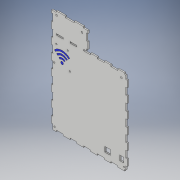
# Autodesk Inventor part: 9 zijplaat met RFID
Saved by Autodesk Inventor 2019 (Build 230136000, 136)
## iProperties
Created: 2021-01-22
Part Number: 9 zijplaat met RFID
Material: Generic
Document SubType Name: Sheet Metal
Designer: Stefan
Density: 1 g/cm^3
Sheet Metal Rule: Default_mm
Appearance: Default
Author: Stefan
Autodesk Inventor part; units mm, degrees
ref_plane "YZ Plane" through (0, 0, 0) normal (1, 0, 0) x (0, 1, 0)
ref_plane "XZ Plane" through (0, 0, 0) normal (0, 1, 0) x (-1, 0, 0)
ref_plane "XY Plane" through (0, 0, 0) normal (0, 0, 1) x (1, 0, 0)
sketch "Sketch1" plane through (0, 0, 0) normal (0, 0, 1) x (1, 0, 0)
  line L0 (-80, -90.5) -> (80, -90.5)
  line L1 (80, -90.5) -> (80, 90.5)
  line L2 (80, 90.5) -> (-80, 90.5)
  line L3 (-80, 90.5) -> (-80, -90.5)
  line L4 (-80, -90.5) -> (80, 90.5) construction
  line L5 (80, -90.5) -> (-80, 90.5) construction
  point P0 (0, 0)
  dimension "d0" = 160
  dimension "d1" = 181
  constraints: 12 end point, 2 midpoint, 2 parallel, 1 horizontal, 1 perpendicular
  measures "d0" distance of L2.end L1.end
  measures "d1" distance of L1.end L0.end
extrude "Extrusion1" add sketch "Sketch1" along normal blind 3
sketch "Sketch2" plane through (0, 0, 3) normal (0, 0, 1) x (1, 0, 0)
  line L0 (80, 90.5) -> (-80, 90.5) projected
  line L1 (-80, 90.5) -> (-72.5, 90.5)
  line L2 (-72.5, 90.5) -> (-72.5, 93.5)
  line L3 (-72.5, 93.5) -> (-80, 93.5)
  line L4 (-80, 93.5) -> (-80, 90.5)
  line L5 (62.5, 90.5) -> (70, 90.5)
  line L6 (70, 90.5) -> (70, 93.5)
  line L7 (70, 93.5) -> (62.5, 93.5)
  line L8 (62.5, 93.5) -> (62.5, 90.5)
  line L9 (-80, -93.5) -> (-72.5, -93.5)
  line L10 (-72.5, -93.5) -> (-72.5, -90.5)
  line L11 (-72.5, -90.5) -> (-80, -90.5)
  line L12 (-80, -90.5) -> (-80, -93.5)
  line L13 (62.5, -93.5) -> (70, -93.5)
  line L14 (70, -93.5) -> (70, -90.5)
  line L15 (70, -90.5) -> (62.5, -90.5)
  line L16 (62.5, -90.5) -> (62.5, -93.5)
  line L17 (-57.5, 90.5) -> (-42.5, 90.5)
  line L18 (-42.5, 90.5) -> (-42.5, 93.5)
  line L19 (-42.5, 93.5) -> (-57.5, 93.5)
  line L20 (-57.5, 93.5) -> (-57.5, 90.5)
  line L21 (-27.5, 90.5) -> (-12.5, 90.5)
  line L22 (-12.5, 93.5) -> (-27.5, 93.5)
  line L23 (-27.5, 93.5) -> (-27.5, 90.5)
  line L24 (-12.5, 90.5) -> (-12.5, 93.5)
  line L25 (2.5, 90.5) -> (17.5, 90.5)
  line L26 (17.5, 93.5) -> (2.5, 93.5)
  line L27 (2.5, 93.5) -> (2.5, 90.5)
  line L28 (17.5, 90.5) -> (17.5, 93.5)
  line L29 (32.5, 90.5) -> (47.5, 90.5)
  line L30 (47.5, 93.5) -> (32.5, 93.5)
  line L31 (32.5, 93.5) -> (32.5, 90.5)
  line L32 (47.5, 90.5) -> (47.5, 93.5)
  line L33 (-57.5, -93.5) -> (-42.5, -93.5)
  line L34 (-42.5, -90.5) -> (-57.5, -90.5)
  line L35 (-57.5, -90.5) -> (-57.5, -93.5)
  line L36 (-42.5, -93.5) -> (-42.5, -90.5)
  line L37 (-27.5, -93.5) -> (-12.5, -93.5)
  line L38 (-12.5, -90.5) -> (-27.5, -90.5)
  line L39 (-27.5, -90.5) -> (-27.5, -93.5)
  line L40 (-12.5, -93.5) -> (-12.5, -90.5)
  line L41 (2.5, -93.5) -> (17.5, -93.5)
  line L42 (17.5, -90.5) -> (2.5, -90.5)
  line L43 (2.5, -90.5) -> (2.5, -93.5)
  line L44 (17.5, -93.5) -> (17.5, -90.5)
  line L45 (32.5, -93.5) -> (47.5, -93.5)
  line L46 (47.5, -90.5) -> (32.5, -90.5)
  line L47 (32.5, -90.5) -> (32.5, -93.5)
  line L48 (47.5, -93.5) -> (47.5, -90.5)
  point P0 (0, 0)
  dimension "d4" = 7.5
  dimension "d5" = 3
  dimension "d8" = 142.5
  dimension "d11" = 184
  dimension "d14" = 15
  dimension "d15" = 3
  dimension "d16" = 15
  dimension "d19" = 30
  dimension "d22" = 184
  constraints: 96 end point, 4 horizontal, 4 parallel, 2 collinear, 2 perpendicular, 2 vertical, 1 point on line, 78 other
  measures "d4" distance of L3.end L2.end
  measures "d5" distance of L2.end L1.end
  measures "d8" distance of L2.end L6.end
  measures "d11" distance of L2.end L10.end
  measures "d14" distance of L19.end L18.end
  measures "d15" distance of L18.end L17.end
  measures "d16" distance between parallel lines of L20 L2
  measures "d19" distance of L17.end L21.end
  measures "d22" distance of L17.end L33.end
extrude "Extrusion2" add sketch "Sketch2" against normal blind 3
sketch "Sketch3" plane through (0, 0, 3) normal (0, 0, 1) x (1, 0, 0)
  line L0 (-80, 93.5) -> (-80, -93.5) projected
  line L1 (-80, 82.5) -> (-83, 82.5)
  line L2 (-83, 82.5) -> (-83, 67.5)
  line L3 (-83, 67.5) -> (-80, 67.5)
  line L4 (-80, 67.5) -> (-80, 82.5)
  line L5 (-80, 52.5) -> (-83, 52.5)
  line L6 (-83, 52.5) -> (-83, 37.5)
  line L7 (-83, 37.5) -> (-80, 37.5)
  line L8 (-80, 37.5) -> (-80, 52.5)
  line L9 (-80, 22.5) -> (-83, 22.5)
  line L10 (-83, 22.5) -> (-83, 7.5)
  line L11 (-83, 7.5) -> (-80, 7.5)
  line L12 (-80, 7.5) -> (-80, 22.5)
  line L13 (-80, -7.5) -> (-83, -7.5)
  line L14 (-83, -7.5) -> (-83, -22.5)
  line L15 (-83, -22.5) -> (-80, -22.5)
  line L16 (-80, -22.5) -> (-80, -7.5)
  line L17 (-80, -37.5) -> (-83, -37.5)
  line L18 (-83, -37.5) -> (-83, -52.5)
  line L19 (-83, -52.5) -> (-80, -52.5)
  line L20 (-80, -52.5) -> (-80, -37.5)
  line L21 (-80, -67.5) -> (-83, -67.5)
  line L22 (-83, -67.5) -> (-83, -82.5)
  line L23 (-83, -82.5) -> (-80, -82.5)
  line L24 (-80, -82.5) -> (-80, -67.5)
  line L25 (83, 82.5) -> (80, 82.5)
  line L26 (80, 82.5) -> (80, 67.5)
  line L27 (80, 67.5) -> (83, 67.5)
  line L28 (83, 67.5) -> (83, 82.5)
  line L29 (83, 52.5) -> (80, 52.5)
  line L30 (80, 52.5) -> (80, 37.5)
  line L31 (80, 37.5) -> (83, 37.5)
  line L32 (83, 37.5) -> (83, 52.5)
  line L33 (83, 22.5) -> (80, 22.5)
  line L34 (80, 22.5) -> (80, 7.5)
  line L35 (80, 7.5) -> (83, 7.5)
  line L36 (83, 7.5) -> (83, 22.5)
  line L37 (83, -7.5) -> (80, -7.5)
  line L38 (80, -7.5) -> (80, -22.5)
  line L39 (80, -22.5) -> (83, -22.5)
  line L40 (83, -22.5) -> (83, -7.5)
  line L41 (83, -37.5) -> (80, -37.5)
  line L42 (80, -37.5) -> (80, -52.5)
  line L43 (80, -52.5) -> (83, -52.5)
  line L44 (83, -52.5) -> (83, -37.5)
  line L45 (83, -67.5) -> (80, -67.5)
  line L46 (80, -67.5) -> (80, -82.5)
  line L47 (80, -82.5) -> (83, -82.5)
  line L48 (83, -82.5) -> (83, -67.5)
  point P0 (0, 0)
  dimension "d27" = 3
  dimension "d28" = 15
  dimension "d29" = 11
  dimension "d32" = 30
  dimension "d35" = 163
  constraints: 96 end point, 2 horizontal, 2 parallel, 1 collinear, 1 perpendicular, 1 point on line, 1 vertical, 87 other
  measures "d27" distance of L3.end L2.end
  measures "d28" distance of L2.end L1.end
  measures "d29" distance from line of L0.start L1
  measures "d32" distance of L1.start L5.start
  measures "d35" distance of L1.start L25.start
extrude "Extrusion3" add sketch "Sketch3" against normal blind 3
sketch "Sketch5" plane through (0, 0, 3) normal (0, 0, 1) x (1, 0, 0)
  line L0 (-79.5, 20.5) -> (-40.5, 20.5) construction
  line L1 (-40.5, 20.5) -> (-40.5, 80.5) construction
  line L2 (-40.5, 80.5) -> (-79.5, 80.5) construction
  line L3 (-79.5, 80.5) -> (-79.5, 20.5) construction
  line L4 (-79.5, 20.5) -> (-40.5, 80.5) construction
  line L5 (-40.5, 20.5) -> (-79.5, 80.5) construction
  circle A0 centre (-72.45, 73.65) radius 1.65
  circle A1 centre (-47.55, 73.65) radius 1.65
  circle A2 centre (-77.15, 36.15) radius 1.65
  circle A3 centre (-42.85, 36.15) radius 1.65
  line L6 (-80, 67.5) -> (-80, 52.5) projected
  line L7 (-57.5, 90.5) -> (-72.5, 90.5) projected
  point P0 (0, 0)
  point P1 (-60, 50.5)
  dimension "d43" = 39
  dimension "d44" = 60
  dimension "d45" = 3.3
  dimension "d46" = 3.3
  dimension "d47" = 3.3
  dimension "d48" = 3.3
  dimension "d49" = 5.4
  dimension "d50" = 5.2
  dimension "d51" = 5.2
  dimension "d52" = 5.4
  dimension "d53" = 0.7
  dimension "d54" = 14
  dimension "d55" = 0.7
  dimension "d56" = 14
  dimension "d57" = 0.5
  dimension "d58" = 10
  constraints: 12 end point, 4 centre point, 2 midpoint, 2 parallel, 1 horizontal, 1 perpendicular
  measures "d43" distance of L2.end L2.start
  measures "d44" distance of L2.start L0.end
  measures "d45" diameter of A0
  measures "d46" diameter of A1
  measures "d47" diameter of A3
  measures "d48" diameter of A2
  measures "d49" distance edge to line of A0 L3
  measures "d50" distance edge to line of A0 L2
  measures "d51" distance edge to line of A1 L2
  measures "d52" distance edge to line of A1 L1
  measures "d53" distance edge to line of A2 L3
  measures "d54" distance edge to line of A2 L0
  measures "d55" distance edge to line of A3 L1
  measures "d56" distance edge to line of A3 L0
  measures "d57" distance between parallel lines of L6 L3
  measures "d58" distance between parallel lines of L7 L2
extrude "Extrusion4" cut sketch "Sketch5" against normal blind 10
sketch "Sketch6" plane through (0, 0, 3) normal (0, 0, 1) x (1, 0, 0)
  line L0 (-71.5024, 68.4241) -> (-38.422, 68.4241) construction
  line L1 (-38.422, 68.4241) -> (-38.422, 39.0388) construction
  line L2 (-38.422, 39.0388) -> (-71.5024, 39.0388) construction
  line L3 (-71.5024, 39.0388) -> (-71.5024, 68.4241) construction
  circle A0 centre (-60, 43.65) radius 3.1114
  line L4 (-60, 43.65) -> (-31.9595, 43.65) construction
  line L5 (-60, 43.65) -> (-31.9595, 43.65) construction
  arc A1 (-55.325, 48.325) -> (-64.675, 48.325) centre (-60, 43.65) ccw
  arc A2 (-50.4247, 53.2253) -> (-69.5753, 53.2253) centre (-60, 43.65) ccw
  arc A3 (-45.4364, 58.2136) -> (-74.5636, 58.2136) centre (-60, 43.65) ccw
  arc A4 (-42.9616, 60.6884) -> (-77.0384, 60.6884) centre (-60, 43.65) ccw
  line L6 (-60, 43.65) -> (-30.904, 43.65) construction
  line L7 (-60, 43.65) -> (-30.904, 43.65) construction
  arc A5 (-52.8996, 50.7504) -> (-67.1004, 50.7504) centre (-60, 43.65) ccw
  arc A6 (-47.9498, 55.7002) -> (-72.0502, 55.7002) centre (-60, 43.65) ccw
  circle A7 centre (-77.15, 36.15) radius 1.65 projected
  circle A8 centre (-72.45, 73.65) radius 1.65 projected
  line L8 (-60, 43.65) -> (-62.2001, 45.8501)
  line L9 (-64.675, 48.325) -> (-67.1004, 50.7504)
  line L10 (-69.5753, 53.2253) -> (-72.0502, 55.7002)
  line L11 (-74.5636, 58.2136) -> (-77.0384, 60.6884)
  line L12 (-60, 43.65) -> (-57.7999, 45.8501)
  line L13 (-55.325, 48.325) -> (-52.8996, 50.7504)
  line L14 (-50.4247, 53.2253) -> (-47.9498, 55.7002)
  line L15 (-45.4364, 58.2136) -> (-42.9616, 60.6884)
  point P0 (0, 0)
  dimension "d220" = 10
  dimension "d72" = 3.5
  dimension "d77" = 3.5
  dimension "d101" = 17.15
  dimension "d106" = 24.096
  dimension "d107" = 17.0415
  dimension "d108" = 13.5415
  dimension "d109" = 10.0415
  dimension "d110" = 6.6114
  dimension "d118" = 33.0804
  dimension "d119" = 24.774
  dimension "d120" = 38.422
  dimension "d127" = 7.518
  dimension "d128" = 6.4625
  dimension "d129" = 6.4625
  dimension "d182" = 0
  dimension "d183" = 0
  dimension "d184" = 0
  dimension "d185" = 0
  dimension "d186" = 0
  dimension "d187" = 0
  dimension "d189" = 45
  dimension "d190" = 73.2916
  constraints: 24 end point, 14 point on circle, 7 centre point, 4 horizontal, 1 parallel, 1 perpendicular, 2 other
  measures "d72" radial gap between concentric circles of A0 A1
  measures "d77" radial gap between concentric circles of A3 A4
  measures "d101" horizontal distance of L4.start A7.centre
  measures "d106" radius of A4
  measures "d107" radius of A6
  measures "d108" radius of A2
  measures "d109" radius of A5
  measures "d110" radius of A1
  measures "d118" distance between parallel lines of L1 L3
  measures "d119" distance between parallel lines of L4 L0
  measures "d120" distance from line of point (0, 0) L1
  measures "d127" distance from line of L6.end L1
  measures "d128" distance from line of L4.end L1
  measures "d129" distance from line of L5.end L1
  measures "d182" distance between parallel lines of L9 L8
  measures "d183" distance between parallel lines of L13 L12
  measures "d184" distance between parallel lines of L9 L10
  measures "d185" distance between parallel lines of L11 L10
  measures "d186" distance between parallel lines of L14 L13
  measures "d187" distance between parallel lines of L15 L14
  measures "d189" angle of L15 L1
  measures "d190" distance from line of point (0, 0) L15
extrude "Extrusion5" add sketch "Sketch6" along normal blind 0.1 contours A0 L8 L12 | L12 L8 A0 | A1 L9 A5 L13 | A2 L10 A6 L14 | A3 L11 A4 L15
sketch "Sketch7" plane through (0, 0, 3) normal (0, 0, 1) x (1, 0, 0)
  line L0 (-80, 93.5) -> (-80, 82.5) projected
  line L1 (-80, 93.5) -> (-6.5, 93.5)
  line L2 (-83, 82.5) -> (-83, 97.5) construction
  line L3 (-83, 97.5) -> (-80, 97.5)
  line L4 (-80, 112.5) -> (-83, 112.5)
  line L5 (-83, 112.5) -> (-83, 97.5)
  line L6 (-80, 93.5) -> (-80, 97.5)
  line L7 (-80, 112.5) -> (-80, 127.5)
  line L8 (-80, 127.5) -> (-83, 127.5)
  line L9 (-83, 127.5) -> (-83, 133.5)
  line L10 (-83, 133.5) -> (-3.5, 133.5)
  line L11 (-3.5, 133.5) -> (-3.5, 93.5) construction
  line L12 (-3.5, 133.5) -> (-3.5, 127.5)
  line L13 (-3.5, 127.5) -> (-6.5, 127.5)
  line L14 (-6.5, 127.5) -> (-6.5, 112.5)
  line L15 (-6.5, 112.5) -> (-3.5, 112.5)
  line L16 (-3.5, 112.5) -> (-3.5, 97.5)
  line L17 (-3.5, 97.5) -> (-6.5, 97.5)
  line L18 (-6.5, 97.5) -> (-6.5, 93.5)
  point P0 (0, 0)
  dimension "d135" = 15
  dimension "d136" = 3
  dimension "d137" = 15
  dimension "d138" = 15
  dimension "d139" = 3
  dimension "d140" = 3
  dimension "d141" = 15
  dimension "d142" = 15
  dimension "d143" = 76.5
  dimension "d144" = 34
  dimension "d145" = 40
  dimension "d146" = 0
  constraints: 36 end point, 6 perpendicular, 6 point on line, 3 horizontal, 3 parallel, 2 vertical
  measures "d135" distance of L2.start L2.end
  measures "d136" distance of L4.end L4.start
  measures "d137" distance of L4.start L3.end
  measures "d138" distance of L4.start L7.end
  measures "d139" distance of L7.end L8.end
  measures "d140" distance of L12.end L13.end
  measures "d141" distance of L13.end L14.end
  measures "d142" distance of L15.end L16.end
  measures "d143" distance between parallel lines of L12 L0
  measures "d144" distance between parallel lines of L13 L1
  measures "d145" distance between parallel lines of L10 L1
  measures "d146" distance from line of L11.end L1
extrude "Extrusion6" add sketch "Sketch7" against normal blind 3
sketch "Sketch8" plane through (0, 0, 3) normal (0, 0, 1) x (1, 0, 0)
  line L0 (-3.5, 133.5) -> (-83, 133.5) projected
  line L1 (-73.25, 133.5) -> (-53.25, 133.5)
  line L2 (-53.25, 133.5) -> (-53.25, 136.5)
  line L3 (-53.25, 136.5) -> (-73.25, 136.5)
  line L4 (-73.25, 136.5) -> (-73.25, 133.5)
  line L5 (-83, 133.5) -> (-83, 127.5) projected
  line L6 (-33.25, 133.5) -> (-13.25, 133.5)
  line L7 (-13.25, 133.5) -> (-13.25, 136.5)
  line L8 (-13.25, 136.5) -> (-33.25, 136.5)
  line L9 (-33.25, 136.5) -> (-33.25, 133.5)
  point P0 (0, 0)
  dimension "d149" = 20
  dimension "d150" = 3
  dimension "d151" = 9.75
  dimension "d154" = 40
  constraints: 16 end point, 2 horizontal, 2 parallel, 1 perpendicular, 1 point on line, 8 other
  measures "d149" distance of L3.end L2.end
  measures "d150" distance of L2.end L1.end
  measures "d151" distance between parallel lines of L4 L5
  measures "d154" distance of L1.start L6.start
extrude "Extrusion7" add sketch "Sketch8" against normal blind 3
sketch "Sketch9" plane through (0, 0, 3) normal (0, 0, 1) x (1, 0, 0)
  line L0 (62.5, 90.5) -> (62.5, 93.5) projected
  line L1 (62.5, 93.5) -> (77.5, 93.5)
  line L2 (77.5, 93.5) -> (77.5, 90.5)
  line L3 (77.5, 90.5) -> (62.5, 90.5)
  line L4 (62.5, 90.5) -> (62.5, 93.5)
  line L5 (62.5, -93.5) -> (62.5, -90.5) projected
  line L6 (62.5, -93.5) -> (77.5, -93.5)
  line L7 (77.5, -93.5) -> (77.5, -90.5)
  line L8 (77.5, -90.5) -> (62.5, -90.5)
  line L9 (62.5, -90.5) -> (62.5, -93.5)
  point P0 (0, 0)
  dimension "d162" = 15
  dimension "d163" = 3
  dimension "d164" = 15
  dimension "d165" = 3
  constraints: 16 end point, 4 parallel, 2 horizontal, 2 perpendicular
  measures "d162" distance of L2.end L3.end
  measures "d163" distance of L1.end L2.end
  measures "d164" distance of L8.end L7.end
  measures "d165" distance of L7.end L6.end
extrude "Extrusion8" add sketch "Sketch9" against normal blind 3
sketch "Sketch10" plane through (0, 0, 3) normal (0, 0, 1) x (1, 0, 0)
  line L0 (-80, -82.5) -> (-80, -93.5) projected
  line L1 (-80, -79) -> (80, -79) construction
  line L2 (80, -90.5) -> (80, -82.5) projected
  line L3 (17.5, -90.5) -> (32.5, -90.5) projected
  line L4 (75.75, -79) -> (66.75, -79)
  line L5 (66.75, -79) -> (66.75, -68)
  line L6 (66.75, -68) -> (75.75, -68)
  line L7 (75.75, -68) -> (75.75, -79)
  line L8 (46.25, -79) -> (34.25, -79)
  line L9 (34.25, -79) -> (34.25, -68)
  line L10 (34.25, -68) -> (46.25, -68)
  line L11 (46.25, -68) -> (46.25, -79)
  point P0 (0, 0)
  dimension "d192" = 11.5
  dimension "d193" = 9
  dimension "d194" = 11
  dimension "d195" = 4.25
  dimension "d196" = 12
  dimension "d197" = 11
  dimension "d198" = 20.5
  constraints: 18 end point, 4 parallel, 4 point on line, 3 horizontal, 2 perpendicular
  measures "d192" distance between parallel lines of L3 L1
  measures "d193" distance of L5.end L6.end
  measures "d194" distance of L4.end L5.end
  measures "d195" distance between parallel lines of L2 L7
  measures "d196" distance of L9.end L10.end
  measures "d197" distance of L8.end L9.end
  measures "d198" distance between parallel lines of L5 L11
extrude "Extrusion9" cut sketch "Sketch10" against normal blind 10
sketch "Sketch11" plane through (0, 0, 3) normal (0, 0, 1) x (1, 0, 0)
  circle A0 centre (-76.5, -86) radius 1.5
  circle A1 centre (76.5, -86) radius 1.5
  line L0 (83, -82.5) -> (83, -67.5) projected
  line L1 (62.5, -93.5) -> (77.5, -93.5) projected
  line L2 (-72.5, -93.5) -> (-80, -93.5) projected
  line L3 (-83, -67.5) -> (-83, -82.5) projected
  point P0 (0, 0)
  dimension "d201" = 3
  dimension "d202" = 3
  dimension "d203" = 6.5
  dimension "d204" = 7.5
  dimension "d205" = 7.5
  dimension "d206" = 6.5
  constraints: 2 centre point
  measures "d201" diameter of A0
  measures "d202" diameter of A1
  measures "d203" distance from line of L0 A1.centre
  measures "d204" distance from line of L1 A1.centre
  measures "d205" distance from line of L2 A0.centre
  measures "d206" distance from line of A0.centre L3
extrude "Extrusion10" cut sketch "Sketch11" against normal blind 10
sketch "Sketch12" plane through (0, 0, 3) normal (0, 0, 1) x (1, 0, 0)
  circle A0 centre (70.5, 81) radius 2
  line L0 (80, 82.5) -> (80, 90.5) projected
  line L1 (62.5, 90.5) -> (47.5, 90.5) projected
  circle A1 centre (-16, 124) radius 2
  line L2 (-3.5, 133.5) -> (-13.25, 133.5) projected
  line L3 (-6.5, 112.5) -> (-6.5, 127.5) projected
  point P0 (0, 0)
  dimension "d209" = 4
  dimension "d210" = 9.5
  dimension "d211" = 9.5
  dimension "d212" = 4
  dimension "d213" = 9.5
  dimension "d214" = 9.5
  constraints: 2 centre point
  measures "d209" diameter of A0
  measures "d210" distance from line of L0 A0.centre
  measures "d211" distance from line of L1 A0.centre
  measures "d212" diameter of A1
  measures "d213" distance from line of L2 A1.centre
  measures "d214" distance from line of L3 A1.centre
extrude "Extrusion11" cut sketch "Sketch12" against normal blind 10
sketch "Sketch13" plane through (0, 0, 3) normal (0, 0, 1) x (1, 0, 0)
  circle A0 centre (-72, 128.5) radius 2
  line L0 (-73.25, 133.5) -> (-83, 133.5) projected
  line L1 (-80, 127.5) -> (-80, 112.5) projected
  point P0 (0, 0)
  dimension "d217" = 4
  dimension "d218" = 5
  dimension "d219" = 8
  constraints: 1 centre point
  measures "d217" diameter of A0
  measures "d218" distance from line of L0 A0.centre
  measures "d219" distance from line of L1 A0.centre
extrude "Extrusion12" cut sketch "Sketch13" against normal blind 10
equation "\"d46\" = d45"
equation "\"d47\" = d45"
equation "\"d48\" = d45"
equation "\"d51\" = d50"
equation "\"d52\" = d49"
equation "\"d55\" = d53"
equation "\"d56\" = d54"
equation "\"d203\" = d206"
equation "\"d204\" = d205"
equation "\"BendRadius\" = Thickness"
equation "\"BendReliefWidth\" = Thickness"
equation "\"BendReliefDepth\" = 0.5 * Thickness"
equation "\"CornerReliefSize\" = 4 * Thickness"
equation "\"MinimumRemnant\" = 2 * Thickness"
equation "\"TransitionRadius\" = BendRadius"
equation "\"JacobiRadiusSize\" = BendRadius"
equation "\"GapSize\" = Thickness"
equation "\"Thickness\" = 0.5"
body "Solid1"
